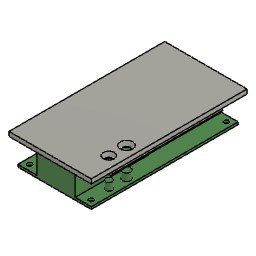
Case v8 (Autodesk Fusion 360 design; units mm, degrees)
Autodesk Fusion 360 part; units mm, degrees
note: some values were not read from the file. Set by a fixed rule: which sketch regions a step uses.
sketch "Sketch1" plane through (0, 0, 0) normal (0, 0, 1) x (1, 0, 0)
  line L0 (25, 50) -> (-25, 50)
  line L1 (-25, 50) -> (-25, -50)
  line L2 (-25, -50) -> (25, -50)
  line L3 (25, -50) -> (25, 50)
  line L4 (25, 50) -> (-25, -50) construction
  line L5 (-25, 50) -> (25, -50) construction
  circle A0 centre (-21, 46) radius 1.6
  line L6 (0, 2.5) -> (0, 20)
  circle A1 centre (21, 46) radius 1.6
  line L7 (20, 0) -> (2.5, 0)
  circle A2 centre (21, -46) radius 1.6
  circle A3 centre (-21, -46) radius 1.6
  dimension "d1" = 50
  dimension "d2" = 100
  dimension "d5" = 3.2
  dimension "d6" = 4
  dimension "d7" = 4
  constraint horizontal L0
  constraint perpendicular L0 L1
  constraint parallel L0 L2
  constraint parallel L1 L3
  constraint coincident L4 origin
  constraint coincident L5 origin
  constraint symmetric A0 L6 A1
  constraint symmetric A0 L7 A3
  constraint symmetric A1 L7 A2
  measures "d1" distance of L1.end L2.end
  measures "d2" distance of L0.end L1.end
  measures "d5" diameter of A0
  measures "d6" distance of L0 A0.centre
  measures "d7" distance of L1 A0.centre
extrude "Extrude1" add sketch "Sketch1" along normal blind 1.6 makes body 1
sketch "Sketch2" plane through (0, 0, 1.6) normal (0, 0, 1) x (-1, 0, 0)
  circle A0 centre (21, -46) radius 1.6
  circle A1 centre (-21, 46) radius 1.6
  circle A2 centre (-21, -46) radius 1.6
  circle A3 centre (21, 46) radius 1.6
  line L0 (-25, 50) -> (-25, -50)
  line L1 (-25, -50) -> (25, -50)
  line L2 (25, -50) -> (25, 50)
  line L3 (25, 50) -> (-25, 50)
  line L4 (7.5, -51.87) -> (-7.5, -51.87)
  line L5 (-7.5, -51.87) -> (-7.5, -33.87)
  line L6 (-7.5, -33.87) -> (7.5, -33.87)
  line L7 (7.5, -33.87) -> (7.5, -51.87)
  dimension "d8" = 15
  dimension "d9" = 18
  dimension "d11" = 1.87
  dimension "d12" = 17.5
  dimension "d68" = 17.5
  constraint horizontal L4
  constraint vertical L5
  constraint horizontal L6
  constraint vertical L7
  measures "d8" distance of L4.start L4.end
  measures "d9" distance of L4.start L6.end
  measures "d11" distance of L1 L4
  measures "d12" distance of L0 L5
  measures "d68" distance of L1.end L7
extrude "Extrude2" add sketch "Sketch2" along normal blind 13 contours L1 L5 L6 L7 | L1 L4 L5 L7 bodies 1
sketch "Sketch3" plane through (0, 0, 1.6) normal (0, 0, 1) x (-1, 0, 0)
  line L0 (7.5, -33.87) -> (7.5, -50)
  line L1 (7.5, -50) -> (25, -50)
  line L2 (25, -50) -> (25, 50)
  line L3 (25, 50) -> (-25, 50)
  line L4 (-25, 50) -> (-25, -50)
  line L5 (-25, -50) -> (-7.5, -50)
  line L6 (-7.5, -50) -> (-7.5, -33.87)
  line L7 (-7.5, -33.87) -> (7.5, -33.87)
  circle A0 centre (21, -46) radius 1.6
  circle A1 centre (-21, 46) radius 1.6
  circle A2 centre (-21, -46) radius 1.6
  circle A3 centre (21, 46) radius 1.6
  line L8 (12, 0) -> (-14, 0)
  line L9 (-14, 0) -> (-14, 50)
  line L10 (-14, 50) -> (12, 50)
  line L11 (12, 50) -> (12, 0)
  dimension "d15" = 13
  dimension "d16" = 26
  dimension "d17" = 50
  dimension "d18" = 11
  constraint horizontal L8
  constraint vertical L9
  constraint horizontal L10
  constraint vertical L11
  constraint collinear L3 L10
  measures "d15" distance of L2 L11
  measures "d16" distance of L9.end L10.end
  measures "d17" distance of L8.start L10.end
  measures "d18" distance of L4 L9
extrude "Extrude3" add sketch "Sketch3" along normal blind 16.4 contours L3 L8 L9 L10 L11 bodies 1
sketch "Sketch4" plane through (0, 0, 0) normal (0, 0, -1) x (1, 0, 0)
  circle A0 centre (-21, -46) radius 1.6
  circle A1 centre (21, 46) radius 1.6
  circle A2 centre (21, -46) radius 1.6
  circle A3 centre (-21, 46) radius 1.6
  line L0 (25, -50) -> (25, 50)
  line L1 (25, 50) -> (-25, 50)
  line L2 (-25, 50) -> (-25, -50)
  line L3 (-25, -50) -> (25, -50)
  line L4 (25.5, -50.5) -> (25.5, 50.5)
  line L5 (25.5, 50.5) -> (-25.5, 50.5)
  line L6 (-25.5, 50.5) -> (-25.5, -50.5)
  line L7 (-25.5, -50.5) -> (25.5, -50.5)
  line L8 (28, -53) -> (28, 53)
  line L9 (28, 53) -> (-28, 53)
  line L10 (-28, 53) -> (-28, -53)
  line L11 (-28, -53) -> (28, -53)
  line L12 (-21, 42.8) -> (-25.5, 42.8)
  line L13 (-17.8, 46) -> (-17.8, 50.5)
  arc A4 (-21, 42.8) -> (-17.8, 46) centre (-21, 46) ccw
  line L14 (20, 0) -> (2.5, 0)
  line L15 (-21, -42.8) -> (-25.5, -42.8)
  arc A5 (-17.8, -46) -> (-21, -42.8) centre (-21, -46) ccw
  line L16 (-17.8, -46) -> (-17.8, -50.5)
  line L17 (0, -2.5) -> (0, -20)
  line L18 (21, 42.8) -> (25.5, 42.8)
  arc A6 (17.8, 46) -> (21, 42.8) centre (21, 46) ccw
  line L19 (17.8, 46) -> (17.8, 50.5)
  line L20 (21, -42.8) -> (25.5, -42.8)
  arc A7 (21, -42.8) -> (17.8, -46) centre (21, -46) ccw
  line L21 (17.8, -46) -> (17.8, -50.5)
  dimension "d21" = 0.5
  dimension "d22" = 3
  constraint coincident L6 L12.end
  constraint tangent L12 A4
  constraint perpendicular L6 L12
  constraint coincident L5 L13.end
  constraint tangent L13 A4
  constraint perpendicular L5 L13
  constraint concentric A3 A4
  constraint symmetric L12.start L14 L15.start
  constraint symmetric L12.end L14 L15.end
  constraint symmetric L13.start L14 A5.start
  constraint symmetric L13.end L14 L16.end
  constraint symmetric A4 L14 A5
  constraint symmetric L12.start L17 L18.start
  constraint symmetric L12.end L17 L18.end
  constraint symmetric L13.start L17 A6.start
  constraint symmetric L13.end L17 L19.end
  constraint symmetric A4 L17 A6
  constraint symmetric L15.start L17 L20.start
  constraint symmetric L15.end L17 L20.end
  constraint symmetric A5.start L17 A7.end
  constraint symmetric A5 L17 A7
  constraint symmetric L16.end L17 L21.end
extrude "Extrude4" add sketch "Sketch4" against normal up to surface (18 mm away) separate body contours L8 L9 L10 L11 makes body 2
extrude "Extrude5" add sketch "Sketch4" along normal blind 3 contours A0 | A1 | A2 | A3 | L0 L3 L20 A7 L21 | L0 L3 L4 L7 L20 L21 | L0 L1 L18 A6 L19 | L0 L1 L4 L5 L18 L19 | L2 L3 L6 L7 L15 L16 | L2 L3 L15 A5 L16 | L1 L2 L12 L13 A4 | L1 L2 L5 L6 L12 L13 | L8 L9 L10 L11 bodies 2
sketch "Sketch5" plane through (0, 0, -3) normal (0, 0, -1) x (1, 0, 0)
  line L0 (25.5, -42.8) -> (21, -42.8)
  arc A0 (21, -42.8) -> (17.8, -46) centre (21, -46) ccw
  line L1 (17.8, -46) -> (17.8, -50.5)
  line L2 (17.8, -50.5) -> (-17.8, -50.5)
  line L3 (-17.8, -50.5) -> (-17.8, -46)
  arc A1 (-17.8, -46) -> (-21, -42.8) centre (-21, -46) ccw
  line L4 (-21, -42.8) -> (-25.5, -42.8)
  line L5 (-25.5, -42.8) -> (-25.5, 42.8)
  line L6 (-25.5, 42.8) -> (-21, 42.8)
  arc A2 (-21, 42.8) -> (-17.8, 46) centre (-21, 46) ccw
  line L7 (-17.8, 46) -> (-17.8, 50.5)
  line L8 (-17.8, 50.5) -> (17.8, 50.5)
  line L9 (25.5, 42.8) -> (25.5, -42.8)
  line L10 (-28, -53) -> (28, -53)
  line L11 (28, -53) -> (28, 53)
  line L12 (28, 53) -> (-28, 53)
  line L13 (-28, 53) -> (-28, -53)
  line L14 (28, 53) -> (-28, 53)
  line L15 (-28, 53) -> (-28, -53)
  line L16 (28, -53) -> (28, 53)
  line L17 (-28, -53) -> (28, -53)
  line L18 (17.8, 50.5) -> (17.8, 46)
  arc A3 (17.8, 46) -> (21, 42.8) centre (21, 46) ccw
  line L19 (21, 42.8) -> (25.5, 42.8)
extrude "Extrude6" add sketch "Sketch5" along normal blind 3 contours L0 A0 L1 L2 L3 A1 L4 L5 L6 A2 L7 L8 L9 L18 A3 L19 | L10 L11 L12 L13 L14 L15 L16 L17 bodies 2
sketch "Sketch6" plane through (0, 53, 0) normal (0, 1, 0) x (-1, 0, 0)
  line L0 (28, 18) -> (-28, 18)
  line L1 (-28, 18) -> (-28, -6)
  line L2 (-28, -6) -> (28, -6)
  line L3 (28, -6) -> (28, 18)
  line L4 (-7.5, 1.6) -> (7.5, 1.6)
  line L5 (7.5, 1.6) -> (7.5, 14.6)
  line L6 (7.5, 14.6) -> (-7.5, 14.6)
  line L7 (-7.5, 14.6) -> (-7.5, 1.6)
  line L8 (8, 1.1) -> (8, 15.1)
  line L9 (8, 15.1) -> (-8, 15.1)
  line L10 (-8, 15.1) -> (-8, 1.1)
  line L11 (-8, 1.1) -> (8, 1.1)
  line L12 (-8, 15.1) -> (-8, 18)
  line L13 (8, 15.1) -> (8, 18)
  dimension "d30" = 0.5
  constraint coincident L0 L12.end
  constraint perpendicular L0 L12
  constraint coincident L0 L13.end
  constraint perpendicular L0 L13
extrude "Extrude7" cut sketch "Sketch6" against normal blind 5 contours L0 L9 L12 L13 | L8 L9 L10 L11 | L4 L5 L6 L7 bodies 2
sketch "Sketch7" plane through (0, 0, 1.6) normal (0, 0, 1) x (-1, 0, 0)
  line L0 (-14, 0) -> (-14, 50)
  line L1 (-14, 50) -> (-25, 50)
  line L2 (-25, 50) -> (-25, -50)
  line L3 (-25, -50) -> (-7.5, -50)
  line L4 (-7.5, -50) -> (-7.5, -33.87)
  line L5 (-7.5, -33.87) -> (7.5, -33.87)
  line L6 (7.5, -33.87) -> (7.5, -50)
  line L7 (7.5, -50) -> (25, -50)
  line L8 (25, -50) -> (25, 50)
  line L9 (25, 50) -> (12, 50)
  line L10 (12, 50) -> (12, 0)
  line L11 (12, 0) -> (-14, 0)
  circle A0 centre (21, -46) radius 1.6
  circle A1 centre (-21, 46) radius 1.6
  circle A2 centre (-21, -46) radius 1.6
  circle A3 centre (21, 46) radius 1.6
  point P0 (21, -46)
  point P1 (-21, -46)
  point P2 (21, 46)
  point P3 (-21, 46)
  constraint coincident P0 A0.centre
  constraint coincident P1 A2.centre
  constraint coincident P2 A3.centre
  constraint coincident P3 A1.centre
hole "Hole1" at (-21, -46, 1.6) at (21, -46, 1.6) at (-21, 46, 1.6) at (21, 46, 1.6) direction (0, 0, -1) diameter 2.9 depth 6 tip angle 180 bodies 2
sketch "Sketch8" plane through (0, 0, 18) normal (0, 0, 1) x (-1, 0, 0)
  line L0 (-8, -53) -> (-8, -50.5)
  line L1 (-8, -50.5) -> (-25.5, -50.5)
  line L2 (-25.5, -50.5) -> (-25.5, 50.5)
  line L3 (-25.5, 50.5) -> (25.5, 50.5)
  line L4 (25.5, 50.5) -> (25.5, -50.5)
  line L5 (25.5, -50.5) -> (8, -50.5)
  line L6 (8, -50.5) -> (8, -53)
  line L7 (8, -53) -> (28, -53)
  line L8 (28, -53) -> (28, 53)
  line L9 (28, 53) -> (-28, 53)
  line L10 (-28, 53) -> (-28, -53)
  line L11 (-28, -53) -> (-8, -53)
  line L12 (28, -53) -> (-28, -53)
  line L13 (-28, -53) -> (-28, 53)
  line L14 (-28, 53) -> (28, 53)
  line L15 (28, 53) -> (28, -53)
  constraint horizontal L12
  constraint vertical L13
  constraint horizontal L14
  constraint vertical L15
  constraint coincident L9.end L10.start
  constraint coincident L7.end L8.start
extrude "Extrude8" add sketch "Sketch8" along normal blind 3 separate body makes body 3
sketch "Sketch9" plane through (0, 0, 18) normal (0, 0, -1) x (1, 0, 0)
  line L0 (28, 53) -> (-28, 53)
  line L1 (-28, 53) -> (-28, -53)
  line L2 (-28, -53) -> (28, -53)
  line L3 (28, -53) -> (28, 53)
  line L4 (-8, -50.5) -> (-8, -53)
  line L5 (8, -53) -> (8, -50.5)
  line L6 (7.8, -53) -> (7.8, -50.5)
  line L7 (-7.8, -50.5) -> (-7.8, -53)
  line L8 (-7.8, -50.5) -> (7.8, -50.5)
  line L9 (7.8, -53) -> (-7.8, -53)
  dimension "d69" = -0.2
  dimension "d70" = -0.2
  constraint perpendicular L6 L8
  constraint perpendicular L7 L9
extrude "Extrude9" add sketch "Sketch9" along normal blind 3 contours L2 L6 L7 L8 L9 bodies 3
sketch "Sketch10" plane through (0, 0, 0) normal (0, 1, 0) x (1, 0, 0)
  line L0 (28, -18) -> (-28, -18)
  line L1 (-28, -18) -> (-28, 6)
  line L2 (-28, 6) -> (28, 6)
  line L3 (28, 6) -> (28, -18)
  line L4 (-28, -18) -> (28, -18)
  line L5 (28, -18) -> (28, -21)
  line L6 (28, -21) -> (-28, -21)
  line L7 (-28, -21) -> (-28, -18)
  line L8 (24, 6) -> (24, -18) construction
  line L9 (24, -18) -> (24, -14)
  line L10 (24, -14) -> (26, -14)
  line L11 (26, -14) -> (27, -15.7321)
  line L12 (26, -14) -> (28, -14) construction
  line L13 (27, -15.7321) -> (26, -17.4641)
  line L14 (27, -15.7321) -> (29, -15.7321) construction
  line L15 (26, -17.4641) -> (25.6906, -18)
  line L16 (24, -18) -> (24.1704, -18)
  line L17 (25.6906, -18) -> (24, -18)
  line L18 (24, -10.1359) -> (27.2309, -15.7321)
  line L19 (27.2309, -15.7321) -> (26.1732, -17.5641)
  line L20 (26.1732, -17.5641) -> (25.8638, -18.1)
  line L21 (25.6906, -18) -> (25.9215, -18)
  line L22 (26, -14) -> (26, -13.6)
  dimension "d44" = 4
  dimension "d45" = 4
  dimension "d46" = 2
  dimension "d47" = 60
  dimension "d48" = 2
  dimension "d49" = 120
  dimension "d50" = 2
  constraint perpendicular L4 L9
  constraint perpendicular L9 L10
  constraint horizontal L12
  constraint horizontal L14
  constraint coincident L4 L15.end
  constraint parallel L13 L15
  constraint coincident L4 L16.end
  constraint perpendicular L9 L16
  constraint parallel L11 L18
  constraint parallel L13 L19
  constraint parallel L15 L20
  constraint coincident L8 L18.start
  constraint coincident L4 L21.end
  constraint coincident L20 L21.end
  constraint coincident L18 L22.end
  constraint perpendicular L10 L22
  measures "d45" distance of L8.end L9.end
  measures "d46" distance of L9.end L10.end
  measures "d47" angle of L11 L12
  measures "d48" distance of L10.end L11.end
  measures "d49" angle of L13 L14
  measures "d50" distance of L11.end L13.end
extrude "Extrude12" add sketch "Sketch10" along normal mid plane 75 contours L0 L4 L9 L10 L11 L13 L15 L16 L17 bodies 3
extrude "Extrude13" cut sketch "Sketch10" along normal mid plane 76 contours L0 L4 L11 L13 L15 L18 L19 L20 L21 L22 | L0 L4 L9 L10 L11 L13 L15 L16 L17 bodies 2
mirror "Mirror1" about plane through (0, 0, 0) normal (1, 0, 0) of "Extrude13"
mirror "Mirror2" about plane through (0, 0, 0) normal (1, 0, 0) of "Extrude12"
sketch "Sketch11" plane through (0, 0, -6) normal (0, 0, -1) x (-1, 0, 0)
  line L0 (27.5, 52.5) -> (-27.5, 52.5)
  line L1 (-27.5, 52.5) -> (-27.5, -52.5)
  line L2 (-27.5, -52.5) -> (27.5, -52.5)
  line L3 (27.5, -52.5) -> (27.5, 52.5)
  line L4 (-19, -40) -> (19, -40) construction
  line L5 (19, -40) -> (19, 40) construction
  line L6 (19, 40) -> (-19, 40) construction
  line L7 (-19, 40) -> (-19, -40) construction
  line L8 (-19, -40) -> (19, 40) construction
  line L9 (19, -40) -> (-19, 40) construction
  line L10 (28, 53) -> (-28, 53)
  line L11 (-28, 53) -> (-28, -53)
  line L12 (-28, -53) -> (28, -53)
  line L13 (28, -53) -> (28, 53)
  point P0 (19, -40)
  point P1 (-19, -40)
  point P2 (-19, 40)
  point P3 (19, 40)
  dimension "d60" = 38
  dimension "d61" = 80
  constraint horizontal L4
  constraint perpendicular L4 L5
  constraint parallel L4 L6
  constraint parallel L5 L7
  constraint coincident L8 origin
  constraint coincident L9 origin
  constraint coincident P0 L4.end
  constraint coincident P1 L4.start
  constraint coincident P2 L6.end
  constraint coincident P3 L5.end
  measures "d60" distance of P3 P2
  measures "d61" distance of P0 P3
hole "Hole2" at (-19, -40, -6) at (19, -40, -6) at (-19, 40, -6) at (19, 40, -6) direction (0, 0, 1) diameter 2.4 depth 2.5 tip angle 180 bodies 2
sketch "Sketch13" plane through (0, 0, 18) normal (0, 0, 1) x (-1, 0, 0)
  line L0 (-8, -53) -> (-8, -50.5)
  line L1 (-8, -50.5) -> (-25.5, -50.5)
  line L2 (-25.5, -50.5) -> (-25.5, -38)
  line L3 (-25.5, 50.5) -> (25.5, 50.5)
  line L4 (25.5, -38) -> (25.5, -50.5)
  line L5 (25.5, -50.5) -> (8, -50.5)
  line L6 (8, -50.5) -> (8, -53)
  line L7 (8, -53) -> (28, -53)
  line L8 (28, -53) -> (28, 53)
  line L9 (28, 53) -> (-28, 53)
  line L10 (-28, 53) -> (-28, -53)
  line L11 (-28, -53) -> (-8, -53)
  line L12 (25.5, -42.8729) -> (28.546, -42.8729)
  line L13 (28.546, -42.8729) -> (28.546, -48.8729)
  line L14 (28.546, -48.8729) -> (25.5, -48.8729)
  line L15 (25.5, -48.8729) -> (25.5, -42.8729)
  line L16 (-20, 0) -> (-2.5, 0)
  line L17 (28.546, 48.8729) -> (25.5, 48.8729)
  line L18 (28.546, 42.8729) -> (28.546, 48.8729)
  line L19 (25.5, 42.8729) -> (28.546, 42.8729)
  line L20 (25.5, 48.8729) -> (25.5, 42.8729)
  line L21 (0, -2.5) -> (0, -20)
  line L22 (-28.546, -48.8729) -> (-25.5, -48.8729)
  line L23 (-25.5, -48.8729) -> (-25.5, -42.8729)
  line L24 (-28.546, -42.8729) -> (-28.546, -48.8729)
  line L25 (-25.5, -42.8729) -> (-28.546, -42.8729)
  line L26 (-25.5, 42.8729) -> (-28.546, 42.8729)
  line L27 (-28.546, 42.8729) -> (-28.546, 48.8729)
  line L28 (-28.546, 48.8729) -> (-25.5, 48.8729)
  line L29 (-25.5, 48.8729) -> (-25.5, 42.8729)
  line L30 (25.9215, -38) -> (25.5, -38)
  line L31 (-25.5, -38) -> (-25.9215, -38)
  line L32 (-25.9215, -38) -> (-25.9215, 38)
  line L33 (-25.9215, 38) -> (-25.5, 38)
  line L34 (-25.5, 38) -> (-25.5, 50.5)
  line L35 (25.5, 50.5) -> (25.5, 38)
  line L36 (25.5, 38) -> (25.9215, 38)
  line L37 (25.9215, 38) -> (25.9215, -38)
  point P0 (-25.5, -50.5)
  point P1 (-28, -53)
  point P2 (-28, 53)
  point P3 (-25.5, -38)
  dimension "d65" = 6
  constraint horizontal L12
  constraint vertical L13
  constraint horizontal L14
  constraint vertical L15
  constraint coincident L4 L12.start
  constraint symmetric L12.start L16 L19.start
  constraint symmetric L12.end L16 L18.start
  constraint symmetric L13.end L16 L17.start
  constraint symmetric L14.end L16 L17.end
  constraint symmetric L4.start L21 P3
  constraint symmetric L4.end L21 P0
  constraint symmetric L7.end L21 P1
  constraint symmetric L8.end L21 P2
  constraint symmetric L12.start L21 L23.end
  constraint symmetric L12.end L21 L24.start
  constraint symmetric L13.end L21 L22.start
  constraint symmetric L14.end L21 L22.end
  constraint symmetric L17.start L21 L27.end
  constraint symmetric L17.end L21 L28.end
  constraint symmetric L18.start L21 L26.end
  constraint symmetric L19.start L21 L26.start
  measures "d65" distance of L12.start L14.end
extrude "Extrude14" cut sketch "Sketch13" against normal blind 1 contours L10 L22 L24 L25 | L2 L10 L22 L23 L25 | L10 L26 L27 L28 | L10 L26 L28 L29 L34 | L8 L17 L18 L19 | L8 L17 L19 L20 L35 | L8 L12 L13 L14 | L4 L8 L12 L14 L15 bodies 2
sketch "Sketch14" plane through (0, 0, 1.6) normal (0, 0, 1) x (-1, 0, 0)
  line L0 (-14, 0) -> (-14, 50)
  line L1 (-14, 50) -> (-25, 50)
  line L2 (-25, 50) -> (-25, -50)
  line L3 (-25, -50) -> (-7.5, -50)
  line L4 (-7.5, -50) -> (-7.5, -33.87)
  line L5 (-7.5, -33.87) -> (7.5, -33.87)
  line L6 (7.5, -33.87) -> (7.5, -50)
  line L7 (7.5, -50) -> (25, -50)
  line L8 (25, -50) -> (25, 50)
  line L9 (25, 50) -> (12, 50)
  line L10 (12, 50) -> (12, 0)
  line L11 (12, 0) -> (-14, 0)
  circle A0 centre (21, -46) radius 1.6
  circle A1 centre (-21, 46) radius 1.6
  circle A2 centre (-21, -46) radius 1.6
  circle A3 centre (21, 46) radius 1.6
  circle A4 centre (-20.25, 33.25) radius 2.25
  circle A5 centre (-20.25, 21.25) radius 2.75
  dimension "d71" = 4.75
  dimension "d72" = 16.75
  dimension "d73" = 4.75
  dimension "d74" = 12
  dimension "d75" = 5.5
  dimension "d76" = 4.5
  measures "d71" distance of L2 A4.centre
  measures "d72" distance of L1 A4.centre
  measures "d73" distance of L2 A5.centre
  measures "d74" distance of A4.centre A5.centre
  measures "d75" diameter of A5
  measures "d76" diameter of A4
extrude "Extrude15" add sketch "Sketch14" along normal blind 5 contours A4 | A5 bodies 1
sketch "Sketch15" plane through (0, 0, 21) normal (0, 0, 1) x (-1, 0, 0)
  line L0 (28, 53) -> (-28, 53)
  line L1 (-28, 53) -> (-28, -53)
  line L2 (-28, -53) -> (28, -53)
  line L3 (28, -53) -> (28, 53)
  circle A0 centre (-20.25, 21.25) radius 2.75
  circle A1 centre (-20.25, 33.25) radius 2.25
  circle A2 centre (-20.25, 33.25) radius 2.25
extrude "Extrude16" cut sketch "Sketch15" against normal blind 7 contours A0 | A1 A2 bodies 3
chamfer "Chamfer1" distance 1.5 distance2 2.5 2 edges at (22.3477, -34.0636, 21) (22.8139, -22.2444, 21) measured on face at (-12.7426, -6.6856, 21) measured on face at (-12.7426, -6.6856, 21) on bodies 3
hidden bodies 2
equation "d19 = 18 mm - 1.6 mm"
named bodies: "PCB", "Lid"
